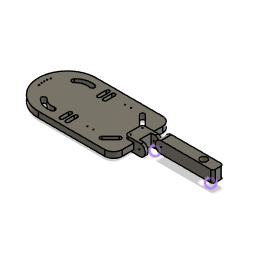
Pratham_Final (Autodesk Fusion 360 design; units mm, degrees)
Autodesk Fusion 360 part; units mm, degrees
sketch "Sketch1" plane through (0, 0, 0) normal (0, 1, 0) x (1, 0, 0)
  line L0 (70, -10) -> (260, -10)
  line L1 (270, -20) -> (270, -100)
  line L2 (260, -110) -> (70, -110)
  arc A0 (260, -110) -> (270, -100) centre (260, -100) ccw
  arc A1 (270, -20) -> (260, -10) centre (260, -20) ccw
  arc A2 (70, -10) -> (70, -110) centre (70, -60) ccw
  arc A3 (78.2923, -29.7488) -> (58.2074, -35.8121) centre (73.4661, -50.0595) ccw
  arc A4 (80.1417, -21.9655) -> (52.3601, -30.3524) centre (73.4661, -50.0595) ccw
  arc A5 (52.3601, -30.3524) -> (58.2074, -35.8121) centre (55.2838, -33.0822) ccw
  arc A6 (78.2923, -29.7488) -> (80.1417, -21.9655) centre (79.217, -25.8571) ccw
  arc A7 (58.5507, -83.6436) -> (78.481, -90.197) centre (74.1537, -69.7742) ccw
  arc A8 (58.5507, -83.6436) -> (52.5714, -88.9585) centre (55.561, -86.301) ccw
  arc A9 (52.5714, -88.9585) -> (80.1392, -98.0232) centre (74.1537, -69.7742) ccw
  arc A10 (80.1392, -98.0232) -> (78.481, -90.197) centre (79.3101, -94.1101) ccw
  circle A11 centre (30, -60) radius 1
  circle A12 centre (30.3163, -54.9793) radius 1
  circle A13 centre (31.268, -50.0083) radius 1
  circle A14 centre (30.3143, -65.0044) radius 1
  circle A15 centre (31.2694, -69.9968) radius 1
  dimension "d6" = 2
  dimension "d7" = 2
  dimension "d8" = 2
  dimension "d9" = 2
  dimension "d10" = 2
  constraint horizontal L0
  constraint vertical L1
  constraint horizontal L2
  constraint tangent A3 A5
  measures "d6" diameter of A11
  measures "d7" diameter of A12
  measures "d8" diameter of A13
  measures "d9" diameter of A14
  measures "d10" diameter of A15
extrude "Extrude1" add sketch "Sketch1" along normal blind 10 makes body 1
sketch "Sketch2" plane through (0, 10, 0) normal (0, 1, 0) x (-1, 0, 0)
  arc A0 (-78.2923, 29.7488) -> (-80.1417, 21.9655) centre (-79.217, 25.8571) ccw
  arc A1 (-78.2923, 29.7488) -> (-58.2074, 35.8121) centre (-73.4661, 50.0595) ccw
  arc A2 (-52.3601, 30.3524) -> (-58.2074, 35.8121) centre (-55.2838, 33.0822) ccw
  arc A3 (-80.1417, 21.9655) -> (-52.3601, 30.3524) centre (-73.4661, 50.0595) ccw
  circle A4 centre (-30.3163, 54.9793) radius 1
  circle A5 centre (-31.2694, 69.9968) radius 1
  arc A6 (-58.5507, 83.6436) -> (-52.5714, 88.9585) centre (-55.561, 86.301) ccw
  arc A7 (-58.5507, 83.6436) -> (-78.481, 90.197) centre (-74.1537, 69.7742) ccw
  arc A8 (-80.1392, 98.0232) -> (-78.481, 90.197) centre (-79.3101, 94.1101) ccw
  arc A9 (-52.5714, 88.9585) -> (-80.1392, 98.0232) centre (-74.1537, 69.7742) ccw
  circle A10 centre (-31.268, 50.0083) radius 1
  circle A11 centre (-30, 60) radius 1
  circle A12 centre (-30.3143, 65.0044) radius 1
  arc A13 (-270, 20) -> (-260, 10) centre (-260, 20) ccw
  line L0 (-260, 10) -> (-70, 10)
  arc A14 (-70, 10) -> (-70, 110) centre (-70, 60) ccw
  line L1 (-70, 110) -> (-260, 110)
  arc A15 (-260, 110) -> (-270, 100) centre (-260, 100) ccw
  line L2 (-270, 100) -> (-270, 20)
  line L3 (-97, 85) -> (-97, 100)
  arc A16 (-97, 100) -> (-103, 100) centre (-100, 100) ccw
  line L4 (-103, 100) -> (-103, 85)
  arc A17 (-103, 85) -> (-97, 85) centre (-100, 85) ccw
  line L5 (-100, 85) -> (-100, 100) construction
  line L6 (-107, 85) -> (-107, 100)
  arc A18 (-107, 100) -> (-113, 100) centre (-110, 100) ccw
  line L7 (-113, 100) -> (-113, 85)
  arc A19 (-113, 85) -> (-107, 85) centre (-110, 85) ccw
  line L8 (-110, 85) -> (-110, 100) construction
  line L9 (-107, 20) -> (-107, 35)
  arc A20 (-107, 35) -> (-113, 35) centre (-110, 35) ccw
  line L10 (-113, 35) -> (-113, 20)
  arc A21 (-113, 20) -> (-107, 20) centre (-110, 20) ccw
  line L11 (-110, 20) -> (-110, 35) construction
  line L12 (-97, 20) -> (-97, 35)
  arc A22 (-97, 35) -> (-103, 35) centre (-100, 35) ccw
  line L13 (-103, 35) -> (-103, 20)
  arc A23 (-103, 20) -> (-97, 20) centre (-100, 20) ccw
  line L14 (-100, 20) -> (-100, 35) construction
  dimension "d13" = 6
  dimension "d14" = 6
  constraint tangent L3 A16
  constraint tangent A16 L4
  constraint parallel L3 L4
  constraint tangent L4 A17
  constraint tangent L3 A17
  constraint vertical L5
  constraint tangent L6 A18
  constraint tangent A18 L7
  constraint parallel L6 L7
  constraint tangent L7 A19
  constraint tangent L6 A19
  constraint parallel L4 L8
  constraint tangent L9 A20
  constraint tangent A20 L10
  constraint parallel L9 L10
  constraint tangent L10 A21
  constraint tangent L9 A21
  constraint vertical L11
  constraint tangent L12 A22
  constraint tangent A22 L13
  constraint parallel L12 L13
  constraint tangent L13 A23
  constraint tangent L12 A23
  constraint vertical L14
  measures "d13" diameter of A20
  measures "d14" diameter of A22
extrude "Extrude2" cut sketch "Sketch2" against normal blind 10 contours L3 A16 L4 A17 | L6 A18 L7 A19 | L9 A20 L10 A21 | L12 A22 L13 A23 bodies 1
sketch "Sketch3" plane through (0, 10, 0) normal (0, 1, 0) x (-1, 0, 0)
  line L0 (-97, 35) -> (-97, 20)
  arc A0 (-103, 20) -> (-97, 20) centre (-100, 20) ccw
  line L1 (-103, 20) -> (-103, 35)
  arc A1 (-97, 35) -> (-103, 35) centre (-100, 35) ccw
  line L2 (-97, 100) -> (-97, 85)
  arc A2 (-103, 85) -> (-97, 85) centre (-100, 85) ccw
  line L3 (-103, 85) -> (-103, 100)
  arc A3 (-97, 100) -> (-103, 100) centre (-100, 100) ccw
  line L4 (-107, 35) -> (-107, 20)
  arc A4 (-113, 20) -> (-107, 20) centre (-110, 20) ccw
  line L5 (-113, 20) -> (-113, 35)
  arc A5 (-107, 35) -> (-113, 35) centre (-110, 35) ccw
  line L6 (-107, 100) -> (-107, 85)
  arc A6 (-113, 85) -> (-107, 85) centre (-110, 85) ccw
  line L7 (-113, 85) -> (-113, 100)
  arc A7 (-107, 100) -> (-113, 100) centre (-110, 100) ccw
  arc A8 (-78.2923, 29.7488) -> (-80.1417, 21.9655) centre (-79.217, 25.8571) ccw
  arc A9 (-78.2923, 29.7488) -> (-58.2074, 35.8121) centre (-73.4661, 50.0595) ccw
  arc A10 (-52.3601, 30.3524) -> (-58.2074, 35.8121) centre (-55.2838, 33.0822) ccw
  arc A11 (-80.1417, 21.9655) -> (-52.3601, 30.3524) centre (-73.4661, 50.0595) ccw
  circle A12 centre (-30.3163, 54.9793) radius 1
  circle A13 centre (-31.2694, 69.9968) radius 1
  arc A14 (-58.5507, 83.6436) -> (-52.5714, 88.9585) centre (-55.561, 86.301) ccw
  arc A15 (-58.5507, 83.6436) -> (-78.481, 90.197) centre (-74.1537, 69.7742) ccw
  arc A16 (-80.1392, 98.0232) -> (-78.481, 90.197) centre (-79.3101, 94.1101) ccw
  arc A17 (-52.5714, 88.9585) -> (-80.1392, 98.0232) centre (-74.1537, 69.7742) ccw
  circle A18 centre (-31.268, 50.0083) radius 1
  circle A19 centre (-30, 60) radius 1
  circle A20 centre (-30.3143, 65.0044) radius 1
  arc A21 (-270, 20) -> (-260, 10) centre (-260, 20) ccw
  line L8 (-260, 10) -> (-70, 10)
  arc A22 (-70, 10) -> (-70, 110) centre (-70, 60) ccw
  line L9 (-70, 110) -> (-260, 110)
  arc A23 (-260, 110) -> (-270, 100) centre (-260, 100) ccw
  line L10 (-270, 100) -> (-270, 20)
  circle A24 centre (-135, 25) radius 1
  circle A25 centre (-145, 25) radius 1
  circle A26 centre (-145, 90) radius 1
  circle A27 centre (-135, 90) radius 1
  dimension "d17" = 2
  dimension "d18" = 2
  dimension "d19" = 2
  dimension "d20" = 2
  measures "d17" diameter of A24
  measures "d18" diameter of A25
  measures "d19" diameter of A26
  measures "d20" diameter of A27
extrude "Extrude3" cut sketch "Sketch3" against normal blind 10 contours A24 | A25 | A26 | A27 bodies 1
sketch "Sketch4" plane through (0, 10, 0) normal (0, 1, 0) x (-1, 0, 0)
  circle A0 centre (-145, 25) radius 1
  circle A1 centre (-145, 90) radius 1
  circle A2 centre (-135, 25) radius 1
  circle A3 centre (-135, 90) radius 1
  line L0 (-97, 35) -> (-97, 20)
  arc A4 (-103, 20) -> (-97, 20) centre (-100, 20) ccw
  line L1 (-103, 20) -> (-103, 35)
  arc A5 (-97, 35) -> (-103, 35) centre (-100, 35) ccw
  line L2 (-97, 100) -> (-97, 85)
  arc A6 (-103, 85) -> (-97, 85) centre (-100, 85) ccw
  line L3 (-103, 85) -> (-103, 100)
  arc A7 (-97, 100) -> (-103, 100) centre (-100, 100) ccw
  line L4 (-107, 35) -> (-107, 20)
  arc A8 (-113, 20) -> (-107, 20) centre (-110, 20) ccw
  line L5 (-113, 20) -> (-113, 35)
  arc A9 (-107, 35) -> (-113, 35) centre (-110, 35) ccw
  line L6 (-107, 100) -> (-107, 85)
  arc A10 (-113, 85) -> (-107, 85) centre (-110, 85) ccw
  line L7 (-113, 85) -> (-113, 100)
  arc A11 (-107, 100) -> (-113, 100) centre (-110, 100) ccw
  arc A12 (-78.2923, 29.7488) -> (-80.1417, 21.9655) centre (-79.217, 25.8571) ccw
  arc A13 (-78.2923, 29.7488) -> (-58.2074, 35.8121) centre (-73.4661, 50.0595) ccw
  arc A14 (-52.3601, 30.3524) -> (-58.2074, 35.8121) centre (-55.2838, 33.0822) ccw
  arc A15 (-80.1417, 21.9655) -> (-52.3601, 30.3524) centre (-73.4661, 50.0595) ccw
  circle A16 centre (-30.3163, 54.9793) radius 1
  circle A17 centre (-31.2694, 69.9968) radius 1
  arc A18 (-58.5507, 83.6436) -> (-52.5714, 88.9585) centre (-55.561, 86.301) ccw
  arc A19 (-58.5507, 83.6436) -> (-78.481, 90.197) centre (-74.1537, 69.7742) ccw
  arc A20 (-80.1392, 98.0232) -> (-78.481, 90.197) centre (-79.3101, 94.1101) ccw
  arc A21 (-52.5714, 88.9585) -> (-80.1392, 98.0232) centre (-74.1537, 69.7742) ccw
  circle A22 centre (-31.268, 50.0083) radius 1
  circle A23 centre (-30, 60) radius 1
  circle A24 centre (-30.3143, 65.0044) radius 1
  arc A25 (-270, 20) -> (-260, 10) centre (-260, 20) ccw
  line L8 (-260, 10) -> (-70, 10)
  arc A26 (-70, 10) -> (-70, 110) centre (-70, 60) ccw
  line L9 (-70, 110) -> (-260, 110)
  arc A27 (-260, 110) -> (-270, 100) centre (-260, 100) ccw
  line L10 (-270, 100) -> (-270, 20)
  line L11 (-200, 60) -> (-200, 25)
  arc A28 (-200, 25) -> (-185, 10) centre (-185, 25) ccw
  line L12 (-200, 60) -> (-200, 95)
  arc A29 (-185, 110) -> (-200, 95) centre (-185, 95) ccw
  constraint perpendicular L8 L11
  constraint tangent L11 A28
  constraint coincident L8 A28.end
  constraint tangent L12 A29
  constraint parallel L11 L12
  constraint coincident L9 A29.start
extrude "Extrude4" cut sketch "Sketch4" against normal blind 10 contours A25 L8 L9 A27 L10 L11 A28 L12 A29 bodies 1
sketch "Sketch5" plane through (0, 10, 0) normal (0, 1, 0) x (-1, 0, 0)
  arc A0 (-200, 25) -> (-185, 10) centre (-185, 25) ccw
  line L0 (-185, 10) -> (-70, 10)
  arc A1 (-70, 10) -> (-70, 110) centre (-70, 60) ccw
  line L1 (-70, 110) -> (-185, 110)
  arc A2 (-185, 110) -> (-200, 95) centre (-185, 95) ccw
  line L2 (-200, 95) -> (-200, 25)
  circle A3 centre (-145, 25) radius 1
  circle A4 centre (-145, 90) radius 1
  circle A5 centre (-135, 25) radius 1
  circle A6 centre (-135, 90) radius 1
  line L3 (-97, 35) -> (-97, 20)
  arc A7 (-103, 20) -> (-97, 20) centre (-100, 20) ccw
  line L4 (-103, 20) -> (-103, 35)
  arc A8 (-97, 35) -> (-103, 35) centre (-100, 35) ccw
  line L5 (-97, 100) -> (-97, 85)
  arc A9 (-103, 85) -> (-97, 85) centre (-100, 85) ccw
  line L6 (-103, 85) -> (-103, 100)
  arc A10 (-97, 100) -> (-103, 100) centre (-100, 100) ccw
  line L7 (-107, 35) -> (-107, 20)
  arc A11 (-113, 20) -> (-107, 20) centre (-110, 20) ccw
  line L8 (-113, 20) -> (-113, 35)
  arc A12 (-107, 35) -> (-113, 35) centre (-110, 35) ccw
  line L9 (-107, 100) -> (-107, 85)
  arc A13 (-113, 85) -> (-107, 85) centre (-110, 85) ccw
  line L10 (-113, 85) -> (-113, 100)
  arc A14 (-107, 100) -> (-113, 100) centre (-110, 100) ccw
  arc A15 (-78.2923, 29.7488) -> (-80.1417, 21.9655) centre (-79.217, 25.8571) ccw
  arc A16 (-78.2923, 29.7488) -> (-58.2074, 35.8121) centre (-73.4661, 50.0595) ccw
  arc A17 (-52.3601, 30.3524) -> (-58.2074, 35.8121) centre (-55.2838, 33.0822) ccw
  arc A18 (-80.1417, 21.9655) -> (-52.3601, 30.3524) centre (-73.4661, 50.0595) ccw
  circle A19 centre (-30.3163, 54.9793) radius 1
  circle A20 centre (-31.2694, 69.9968) radius 1
  arc A21 (-58.5507, 83.6436) -> (-52.5714, 88.9585) centre (-55.561, 86.301) ccw
  arc A22 (-58.5507, 83.6436) -> (-78.481, 90.197) centre (-74.1537, 69.7742) ccw
  arc A23 (-80.1392, 98.0232) -> (-78.481, 90.197) centre (-79.3101, 94.1101) ccw
  arc A24 (-52.5714, 88.9585) -> (-80.1392, 98.0232) centre (-74.1537, 69.7742) ccw
  circle A25 centre (-31.268, 50.0083) radius 1
  circle A26 centre (-30, 60) radius 1
  circle A27 centre (-30.3143, 65.0044) radius 1
  line L11 (-167.5, 97.5) -> (-182.5, 82.5)
  arc A28 (-182.5, 82.5) -> (-177.5, 77.5) centre (-180, 80) ccw
  line L12 (-177.5, 77.5) -> (-162.5, 92.5)
  arc A29 (-162.5, 92.5) -> (-167.5, 97.5) centre (-165, 95) ccw
  line L13 (-165, 95) -> (-180, 80) construction
  line L14 (-162.5251, 27.4749) -> (-177.5251, 42.4749)
  arc A30 (-177.5251, 42.4749) -> (-182.4749, 37.5251) centre (-180, 40) ccw
  line L15 (-182.4749, 37.5251) -> (-167.4749, 22.5251)
  arc A31 (-167.4749, 22.5251) -> (-162.5251, 27.4749) centre (-165, 25) ccw
  line L16 (-165, 25) -> (-180, 40) construction
  dimension "d25" = 7
  constraint tangent L11 A28
  constraint tangent A28 L12
  constraint parallel L11 L12
  constraint tangent L12 A29
  constraint tangent L11 A29
  constraint tangent L14 A30
  constraint tangent A30 L15
  constraint parallel L14 L15
  constraint tangent L15 A31
  constraint tangent L14 A31
  constraint perpendicular L12 L16
  measures "d25" diameter of A30
extrude "Extrude5" cut sketch "Sketch5" against normal blind 10 contours L11 A28 L12 A29 | L14 A30 L15 A31 bodies 1
sketch "Sketch6" plane through (0, 10, 0) normal (0, 1, 0) x (-1, 0, 0)
  line L0 (-182.5, 82.5) -> (-167.5, 97.5)
  arc A0 (-162.5, 92.5) -> (-167.5, 97.5) centre (-165, 95) ccw
  line L1 (-162.5, 92.5) -> (-177.5, 77.5)
  arc A1 (-182.5, 82.5) -> (-177.5, 77.5) centre (-180, 80) ccw
  line L2 (-177.5251, 42.4749) -> (-162.5251, 27.4749)
  arc A2 (-167.4749, 22.5251) -> (-162.5251, 27.4749) centre (-165, 25) ccw
  line L3 (-167.4749, 22.5251) -> (-182.4749, 37.5251)
  arc A3 (-177.5251, 42.4749) -> (-182.4749, 37.5251) centre (-180, 40) ccw
  arc A4 (-200, 25) -> (-185, 10) centre (-185, 25) ccw
  line L4 (-185, 10) -> (-70, 10)
  arc A5 (-70, 10) -> (-70, 110) centre (-70, 60) ccw
  line L5 (-70, 110) -> (-185, 110)
  arc A6 (-185, 110) -> (-200, 95) centre (-185, 95) ccw
  line L6 (-200, 95) -> (-200, 25)
  circle A7 centre (-145, 25) radius 1
  circle A8 centre (-145, 90) radius 1
  circle A9 centre (-135, 25) radius 1
  circle A10 centre (-135, 90) radius 1
  line L7 (-97, 35) -> (-97, 20)
  arc A11 (-103, 20) -> (-97, 20) centre (-100, 20) ccw
  line L8 (-103, 20) -> (-103, 35)
  arc A12 (-97, 35) -> (-103, 35) centre (-100, 35) ccw
  line L9 (-97, 100) -> (-97, 85)
  arc A13 (-103, 85) -> (-97, 85) centre (-100, 85) ccw
  line L10 (-103, 85) -> (-103, 100)
  arc A14 (-97, 100) -> (-103, 100) centre (-100, 100) ccw
  line L11 (-107, 35) -> (-107, 20)
  arc A15 (-113, 20) -> (-107, 20) centre (-110, 20) ccw
  line L12 (-113, 20) -> (-113, 35)
  arc A16 (-107, 35) -> (-113, 35) centre (-110, 35) ccw
  line L13 (-107, 100) -> (-107, 85)
  arc A17 (-113, 85) -> (-107, 85) centre (-110, 85) ccw
  line L14 (-113, 85) -> (-113, 100)
  arc A18 (-107, 100) -> (-113, 100) centre (-110, 100) ccw
  arc A19 (-78.2923, 29.7488) -> (-80.1417, 21.9655) centre (-79.217, 25.8571) ccw
  arc A20 (-78.2923, 29.7488) -> (-58.2074, 35.8121) centre (-73.4661, 50.0595) ccw
  arc A21 (-52.3601, 30.3524) -> (-58.2074, 35.8121) centre (-55.2838, 33.0822) ccw
  arc A22 (-80.1417, 21.9655) -> (-52.3601, 30.3524) centre (-73.4661, 50.0595) ccw
  circle A23 centre (-30.3163, 54.9793) radius 1
  circle A24 centre (-31.2694, 69.9968) radius 1
  arc A25 (-58.5507, 83.6436) -> (-52.5714, 88.9585) centre (-55.561, 86.301) ccw
  arc A26 (-58.5507, 83.6436) -> (-78.481, 90.197) centre (-74.1537, 69.7742) ccw
  arc A27 (-80.1392, 98.0232) -> (-78.481, 90.197) centre (-79.3101, 94.1101) ccw
  arc A28 (-52.5714, 88.9585) -> (-80.1392, 98.0232) centre (-74.1537, 69.7742) ccw
  circle A29 centre (-31.268, 50.0083) radius 1
  circle A30 centre (-30, 60) radius 1
  circle A31 centre (-30.3143, 65.0044) radius 1
  circle A32 centre (-190, 50) radius 1
  circle A33 centre (-190, 70) radius 1
  dimension "d28" = 2
  dimension "d29" = 2
  measures "d28" diameter of A32
  measures "d29" diameter of A33
extrude "Extrude6" cut sketch "Sketch6" against normal blind 10 contours A32 | A33 bodies 1
sketch "Sketch7" plane through (0, 0, 0) normal (0, 1, 0) x (1, 0, 0)
  line L0 (235.6116, -42.378) -> (255.6116, -42.378)
  line L1 (255.6116, -42.378) -> (255.6116, -72.378)
  line L2 (255.6116, -72.378) -> (235.6116, -72.378)
  line L3 (235.6116, -72.378) -> (235.6116, -42.378)
extrude "Extrude7" add sketch "Sketch7" along normal blind 20 separate body makes body 2
sketch "Sketch8" plane through (235.6116, 0, 0) normal (-1, 0, 0) x (0, 0, 1)
  line L0 (42.378, 0) -> (72.378, 0)
  line L1 (72.378, 0) -> (72.378, 20)
  line L2 (72.378, 20) -> (42.378, 20)
  line L3 (42.378, 20) -> (42.378, 0)
  line L4 (42.378, 20) -> (72.378, 20)
  line L5 (72.378, 20) -> (72.378, 15)
  line L6 (72.378, 15) -> (42.378, 15)
  line L7 (42.378, 15) -> (42.378, 20)
  line L8 (42.378, 0) -> (72.378, 0)
  line L9 (72.378, 0) -> (72.378, 5)
  line L10 (72.378, 5) -> (42.378, 5)
  line L11 (42.378, 5) -> (42.378, 0)
  dimension "d36" = 5
  dimension "d37" = 5
  constraint horizontal L4
  constraint vertical L5
  constraint horizontal L6
  constraint vertical L7
  constraint coincident L2.end L3.start
  constraint horizontal L8
  constraint vertical L9
  constraint horizontal L10
  constraint vertical L11
  constraint coincident L0.start L3.end
  measures "d36" distance of L2.end L6.end
  measures "d37" distance of L0.start L10.end
extrude "Extrude8" cut sketch "Sketch8" against normal blind 15 contours L1 L3 L6 L10 bodies 2
sketch "Sketch9" plane through (0, 20, 0) normal (0, 1, 0) x (-1, 0, 0)
  line L0 (-235.6116, 72.378) -> (-255.6116, 72.378)
  line L1 (-255.6116, 72.378) -> (-255.6116, 42.378)
  line L2 (-255.6116, 42.378) -> (-235.6116, 42.378)
  line L3 (-235.6116, 42.378) -> (-235.6116, 72.378)
  arc A0 (-235.6116, 67.378) -> (-240.6116, 72.378) centre (-240.6116, 67.378) ccw
  arc A1 (-240.6116, 42.378) -> (-235.6116, 47.378) centre (-240.6116, 47.378) ccw
  dimension "d40" = 5
  dimension "d41" = 5
  constraint coincident L3 A1.end
  constraint coincident L2 A1.start
  measures "d40" distance of L0.start A0.end
  measures "d41" distance of L0.start A0.start
extrude "Extrude9" cut sketch "Sketch9" against normal blind 20 contours L0 L3 A0 | L2 L3 A1 bodies 2
sketch "Sketch10" plane through (0, 20, 0) normal (0, 1, 0) x (-1, 0, 0)
  arc A0 (-235.6116, 67.378) -> (-240.6116, 72.378) centre (-240.6116, 67.378) ccw
  line L0 (-240.6116, 72.378) -> (-255.6116, 72.378)
  line L1 (-255.6116, 72.378) -> (-255.6116, 42.378)
  line L2 (-255.6116, 42.378) -> (-240.6116, 42.378)
  arc A1 (-240.6116, 42.378) -> (-235.6116, 47.378) centre (-240.6116, 47.378) ccw
  line L3 (-235.6116, 47.378) -> (-235.6116, 67.378)
  circle A2 centre (-240.6116, 67.378) radius 1
  circle A3 centre (-240.6116, 47.378) radius 1
  dimension "d50" = 2
  dimension "d51" = 2
  constraint concentric A0 A2
  constraint concentric A1 A3
  measures "d50" diameter of A2
  measures "d51" diameter of A3
extrude "Extrude10" cut sketch "Sketch10" against normal blind 20 contours A2 | A3 bodies 2
sketch "Sketch11" plane through (0, 0, 72.378) normal (0, 0, 1) x (1, 0, 0)
  line L0 (240.6116, 5) -> (240.6116, 0)
  line L1 (240.6116, 0) -> (255.6116, 0)
  line L2 (255.6116, 0) -> (255.6116, 20)
  line L3 (255.6116, 20) -> (240.6116, 20)
  line L4 (240.6116, 20) -> (240.6116, 15)
  line L5 (240.6116, 15) -> (250.6116, 15)
  line L6 (250.6116, 15) -> (250.6116, 5)
  line L7 (250.6116, 5) -> (240.6116, 5)
  line L8 (255.6116, 20) -> (263.1116, 20)
  line L9 (263.1116, 0) -> (255.6116, 0)
  line L10 (255.6116, 0) -> (255.6116, 20)
  arc A0 (263.1116, 0) -> (263.1116, 20) centre (260.195, 10) ccw
  dimension "d55" = 20
  constraint horizontal L8
  constraint horizontal L9
  constraint vertical L10
  constraint coincident L2.end L3.start
  measures "d55" distance of L2.end L1.end
extrude "Extrude11" add sketch "Sketch11" against normal blind 30 contours L2 L8 L9 L10 A0 bodies 2
sketch "Sketch12" plane through (0, 20, 0) normal (0, 1, 0) x (-1, 0, 0)
  circle A0 centre (-240.6116, 67.378) radius 1
  circle A1 centre (-240.6116, 47.378) radius 1
  arc A2 (-235.6116, 67.378) -> (-240.6116, 72.378) centre (-240.6116, 67.378) ccw
  line L0 (-240.6116, 72.378) -> (-263.1116, 72.378)
  line L1 (-263.1116, 42.378) -> (-240.6116, 42.378)
  arc A3 (-240.6116, 42.378) -> (-235.6116, 47.378) centre (-240.6116, 47.378) ccw
  line L2 (-235.6116, 47.378) -> (-235.6116, 67.378)
  line L3 (-270.6116, 67.378) -> (-255.6116, 67.378)
  line L4 (-270.6116, 67.378) -> (-270.6116, 47.378)
  line L5 (-270.6116, 47.378) -> (-255.6116, 47.378)
  line L6 (-255.6116, 47.378) -> (-255.6116, 67.378)
  constraint horizontal L3
  constraint vertical L4
  constraint horizontal L5
  constraint vertical L6
extrude "Extrude12" cut sketch "Sketch12" against normal blind 20 contours L3 L4 L5 L6 bodies 2
sketch "Sketch13" plane through (0, 0, 72.378) normal (0, 0, 1) x (1, 0, 0)
  line L0 (240.6116, 5) -> (240.6116, 0)
  line L1 (240.6116, 0) -> (263.1116, 0)
  arc A0 (263.1116, 0) -> (263.1116, 20) centre (260.195, 10) ccw
  line L2 (263.1116, 20) -> (240.6116, 20)
  line L3 (240.6116, 20) -> (240.6116, 15)
  line L4 (240.6116, 15) -> (250.6116, 15)
  line L5 (250.6116, 15) -> (250.6116, 5)
  line L6 (250.6116, 5) -> (240.6116, 5)
  line L7 (250.6116, 10) -> (260.195, 10)
  constraint midpoint L5 L7.start
  constraint coincident A0.centre L7.end
hole "Hole1" at (260.195, 10, 72.378) direction (0, 0, -1) diameter 2 depth 36 tip angle 118 bodies 2
extrude "Extrude13" cut 1 faces at (247.5537, 5, 54.2324) along direction (0, -1, 0) blind 0.5 on bodies 2 bodies 2
extrude "Extrude14" cut 1 faces at (247.5537, 15, 54.2324) along direction (0, 1, 0) blind 0.5 on bodies 2 bodies 2
move_body "Move1" bodies 2 to x (1, 0, 0) y (0, 1, 0) z (0, 0, 1) at (-50.7556, -5.1027, 2.5484)
sketch "Sketch14" plane through (0, 10, 0) normal (0, 1, 0) x (-1, 0, 0)
  circle A0 centre (-190, 70) radius 1
  circle A1 centre (-190, 50) radius 1
  line L0 (-182.5, 82.5) -> (-167.5, 97.5)
  arc A2 (-162.5, 92.5) -> (-167.5, 97.5) centre (-165, 95) ccw
  line L1 (-162.5, 92.5) -> (-177.5, 77.5)
  arc A3 (-182.5, 82.5) -> (-177.5, 77.5) centre (-180, 80) ccw
  line L2 (-177.5251, 42.4749) -> (-162.5251, 27.4749)
  arc A4 (-167.4749, 22.5251) -> (-162.5251, 27.4749) centre (-165, 25) ccw
  line L3 (-167.4749, 22.5251) -> (-182.4749, 37.5251)
  arc A5 (-177.5251, 42.4749) -> (-182.4749, 37.5251) centre (-180, 40) ccw
  arc A6 (-200, 25) -> (-185, 10) centre (-185, 25) ccw
  line L4 (-185, 10) -> (-70, 10)
  arc A7 (-70, 10) -> (-70, 110) centre (-70, 60) ccw
  line L5 (-70, 110) -> (-185, 110)
  arc A8 (-185, 110) -> (-200, 95) centre (-185, 95) ccw
  line L6 (-200, 95) -> (-200, 25)
  circle A9 centre (-145, 25) radius 1
  circle A10 centre (-145, 90) radius 1
  circle A11 centre (-135, 25) radius 1
  circle A12 centre (-135, 90) radius 1
  line L7 (-97, 35) -> (-97, 20)
  arc A13 (-103, 20) -> (-97, 20) centre (-100, 20) ccw
  line L8 (-103, 20) -> (-103, 35)
  arc A14 (-97, 35) -> (-103, 35) centre (-100, 35) ccw
  line L9 (-97, 100) -> (-97, 85)
  arc A15 (-103, 85) -> (-97, 85) centre (-100, 85) ccw
  line L10 (-103, 85) -> (-103, 100)
  arc A16 (-97, 100) -> (-103, 100) centre (-100, 100) ccw
  line L11 (-107, 35) -> (-107, 20)
  arc A17 (-113, 20) -> (-107, 20) centre (-110, 20) ccw
  line L12 (-113, 20) -> (-113, 35)
  arc A18 (-107, 35) -> (-113, 35) centre (-110, 35) ccw
  line L13 (-107, 100) -> (-107, 85)
  arc A19 (-113, 85) -> (-107, 85) centre (-110, 85) ccw
  line L14 (-113, 85) -> (-113, 100)
  arc A20 (-107, 100) -> (-113, 100) centre (-110, 100) ccw
  arc A21 (-78.2923, 29.7488) -> (-80.1417, 21.9655) centre (-79.217, 25.8571) ccw
  arc A22 (-78.2923, 29.7488) -> (-58.2074, 35.8121) centre (-73.4661, 50.0595) ccw
  arc A23 (-52.3601, 30.3524) -> (-58.2074, 35.8121) centre (-55.2838, 33.0822) ccw
  arc A24 (-80.1417, 21.9655) -> (-52.3601, 30.3524) centre (-73.4661, 50.0595) ccw
  circle A25 centre (-30.3163, 54.9793) radius 1
  circle A26 centre (-31.2694, 69.9968) radius 1
  arc A27 (-58.5507, 83.6436) -> (-52.5714, 88.9585) centre (-55.561, 86.301) ccw
  arc A28 (-58.5507, 83.6436) -> (-78.481, 90.197) centre (-74.1537, 69.7742) ccw
  arc A29 (-80.1392, 98.0232) -> (-78.481, 90.197) centre (-79.3101, 94.1101) ccw
  arc A30 (-52.5714, 88.9585) -> (-80.1392, 98.0232) centre (-74.1537, 69.7742) ccw
  circle A31 centre (-31.268, 50.0083) radius 1
  circle A32 centre (-30, 60) radius 1
  circle A33 centre (-30.3143, 65.0044) radius 1
  line L15 (-230, 50) -> (-326, 50)
  line L16 (-330, 54) -> (-330, 64)
  line L17 (-326, 68) -> (-230, 68)
  line L18 (-230, 68) -> (-230, 50)
  circle A34 centre (-305, 59) radius 6
  arc A35 (-326, 68) -> (-330, 64) centre (-326, 64) ccw
  arc A36 (-330, 54) -> (-326, 50) centre (-326, 54) ccw
  constraint horizontal L15
  constraint vertical L16
  constraint horizontal L17
  constraint vertical L18
  constraint tangent L16 A36
  constraint tangent L16 A35
extrude "Extrude15" add sketch "Sketch14" along normal blind 20 separate body contours L15 L16 L17 L18 A35 A36 makes body 3
sketch "Sketch15" plane through (0, 0, 68) normal (0, 0, 1) x (1, 0, 0)
  line L0 (326, 10) -> (326, 30)
  line L1 (326, 30) -> (230, 30)
  line L2 (230, 30) -> (230, 10)
sketch "Sketch16" plane through (0, 0, 68) normal (0, 0, 1) x (1, 0, 0)
  line L0 (240, 30) -> (230, 30)
  line L1 (230, 30) -> (230, 10)
  line L2 (230, 10) -> (240, 10)
  arc A0 (240, 30) -> (240, 10) centre (240, 20) ccw
  constraint horizontal L0
  constraint vertical L1
  constraint horizontal L2
extrude "Extrude16" cut sketch "Sketch16" against normal blind 18 bodies 3
sketch "Sketch17" plane through (0, 0, 68) normal (0, 0, 1) x (1, 0, 0)
  line L0 (230, 20) -> (240, 20)
  constraint horizontal L0
hole "Hole2" at (240, 20, 68) direction (0, 0, -1) diameter 2 depth 18 tip angle 118 bodies 3
